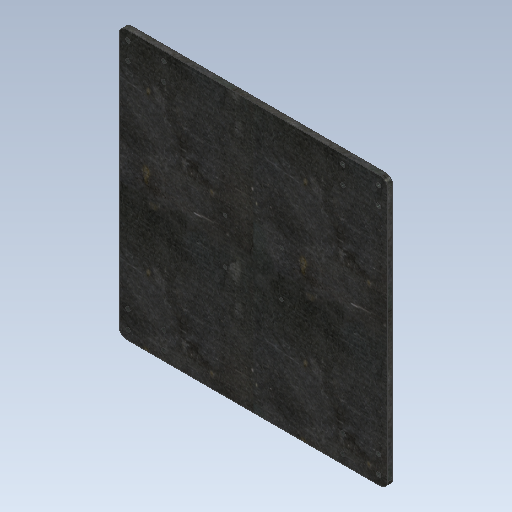
# Autodesk Inventor part: BaseC_1
Saved by Autodesk Inventor 2021.1 (Build 251245010, 245A)
## iProperties
Created: 2023-10-20
Part Number: BaseC_1
Material: Steel
Document SubType Name: Modeling
Designer: user
Density: 7.85 g/cm^3
Appearance: Plate
Mass: 4219.25 g
Surface Area: 1880.88 cm^2
Volume: 537.484 cm^3
Author: user
Autodesk Inventor part; units mm, degrees
ref_plane "YZ Plane" through (0, 0, 0) normal (1, 0, 0) x (0, 1, 0)
ref_plane "XZ Plane" through (0, 0, 0) normal (0, 1, 0) x (-1, 0, 0)
ref_plane "XY Plane" through (0, 0, 0) normal (0, 0, 1) x (1, 0, 0)
sketch "Sketch1" plane through (0, 0, 0) normal (0, 0, 1) x (1, 0, 0)
  line L0 (0, 0) -> (300, 0)
  line L1 (300, 0) -> (300, -300)
  line L2 (300, -300) -> (0, -300)
  line L3 (0, -300) -> (0, 0)
  circle A0 centre (118.5, -125) radius 2
  circle A1 centre (118.5, -175) radius 2
  circle A2 centre (181.5, -175) radius 2
  circle A3 centre (181.5, -125) radius 2
  line L4 (118.5, -125) -> (118.5, -175)
  line L5 (118.5, -125) -> (181.5, -125)
  line L6 (118.5, -175) -> (181.5, -175)
  line L7 (181.5, -125) -> (181.5, -175)
  circle A4 centre (290, -10) radius 2.5
  circle A5 centre (290, -30) radius 2.5
  circle A6 centre (250, -30) radius 2.5
  circle A7 centre (250, -10) radius 2.5
  line L8 (300, -6.9) -> (223, -6.9)
  line L9 (300, -13.1) -> (223, -13.1)
  line L10 (300, -33.1) -> (223, -33.1)
  line L11 (300, -26.9) -> (223, -26.9)
  line L12 (300, -40) -> (222.6975, -40)
  line L13 (240, 0) -> (240, -40)
  circle A8 centre (290, -270) radius 2.5
  circle A9 centre (290, -290) radius 2.5
  circle A10 centre (250, -290) radius 2.5
  circle A11 centre (250, -270) radius 2.5
  circle A12 centre (50, -270) radius 2.5
  circle A13 centre (50, -290) radius 2.5
  circle A14 centre (10, -290) radius 2.5
  circle A15 centre (10, -270) radius 2.5
  circle A16 centre (50, -10) radius 2.5
  circle A17 centre (50, -30) radius 2.5
  circle A18 centre (10, -30) radius 2.5
  circle A19 centre (10, -10) radius 2.5
  dimension "d29" = 50
  dimension "d31" = 50
  dimension "d33" = 300
  dimension "d34" = 300
  dimension "d35" = 118.5
  dimension "d36" = 125
  dimension "d37" = 63
  dimension "d38" = 5
  dimension "d39" = 5
  dimension "d40" = 5
  dimension "d41" = 5
  dimension "d42" = 6.2
  dimension "d43" = 6.9
  dimension "d44" = 10
  dimension "d45" = 10
  dimension "d46" = 10
  dimension "d47" = 10
  dimension "d48" = 10
  dimension "d49" = 40
  dimension "d50" = 40
  dimension "d51" = 10
  dimension "d58" = 10
  dimension "d59" = 40
  dimension "d60" = 5
  dimension "d61" = 5
  dimension "d62" = 5
  dimension "d63" = 5
  dimension "d64" = 40
  dimension "d65" = 40
  dimension "d66" = 5
  dimension "d67" = 5
  dimension "d68" = 5
  dimension "d69" = 5
  dimension "d70" = 40
  dimension "d71" = 40
  dimension "d72" = 5
  dimension "d73" = 5
  dimension "d74" = 5
  dimension "d75" = 5
  dimension "d76" = 40
  dimension "d77" = 40
  constraints: 28 end point, 20 centre point, 8 horizontal, 3 point on line, 2 parallel, 2 perpendicular, 2 vertical, 8 other
  measures "d29" distance of L4.start L4.end
  measures "d31" distance of L5.end L6.end
  measures "d33" distance of L2.end L0.start
  measures "d34" distance of L0.start L0.end
  measures "d35" distance from line of L3 L4.end
  measures "d36" distance from line of L0 L4.start
  measures "d37" distance of L4.start L5.end
  measures "d38" diameter of A4
  measures "d39" diameter of A5
  measures "d40" diameter of A6
  measures "d41" diameter of A7
  measures "d42" distance between parallel lines of L9 L8
  measures "d43" distance between parallel lines of L8 L0
  measures "d44" distance from line of A4.centre L0
  measures "d45" distance from line of A4.centre L1
  measures "d46" distance from line of L1 A5.centre
  measures "d47" distance from line of L12 A5.centre
  measures "d48" distance from line of L0 A7.centre
  measures "d49" distance of A4.centre A7.centre
  measures "d50" distance of A5.centre A6.centre
  measures "d51" distance from line of L12 A6.centre
  measures "d58" distance from line of L13 A7.centre
  measures "d59" distance between parallel lines of L0 L12
  measures "d60" diameter of A8
  measures "d61" diameter of A9
  measures "d62" diameter of A10
  measures "d63" diameter of A11
  measures "d64" distance of A8.centre A11.centre
  measures "d65" distance of A9.centre A10.centre
  measures "d66" diameter of A12
  measures "d67" diameter of A13
  measures "d68" diameter of A14
  measures "d69" diameter of A15
  measures "d70" distance of A12.centre A15.centre
  measures "d71" distance of A13.centre A14.centre
  measures "d72" diameter of A16
  measures "d73" diameter of A17
  measures "d74" diameter of A18
  measures "d75" diameter of A19
  measures "d76" distance of A16.centre A19.centre
  measures "d77" distance of A17.centre A18.centre
extrude "Extrusion1" add sketch "Sketch1" along normal blind 6 contours L0 L13 L12 L1 L2 L3 | L0 L1 L8 L13 | L8 L1 L9 L13 | L9 L1 L11 L13 | L12 L13 L10 L1 | L11 L1 L10 L13 | L5 A3 L7 A2 L6 A1 L4 A0
fillet "Fillet1" radius 8 4 edges at (0, -300, 3) (300, -300, 3) (300, 0, 3) (0, 0, 3)
equation "\"d29\" = d31"
equation "\"d35\" = -0.5 * d37 + 0.5 * d34"
equation "\"d36\" = -0.5 * d29 + 0.5 * d33"
equation "\"d39\" = d38"
equation "\"d40\" = d38"
equation "\"d41\" = d38"
equation "\"d18\" = -0.5 * d12 + 0.5 * d1"
equation "\"d12\" = 74"
equation "\"d1\" = 170"
body "Solid1"
